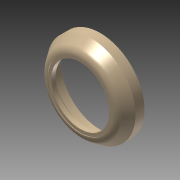
# Autodesk Inventor part: body
Saved by Autodesk Inventor 2015 SP1 (Build 190203100, 203)
## iProperties
Created: 2015-02-16
Part Number: body
Material: Polyethylene, Low Density
Document SubType Name: Modeling
Designer: Jostein
Density: 0.894 g/cm^3
Appearance: Smooth - Off-White
Author: Jostein
Autodesk Inventor part; units mm, degrees
ref_plane "YZ Plane" through (0, 0, 0) normal (1, 0, 0) x (0, 1, 0)
ref_plane "XZ Plane" through (0, 0, 0) normal (0, 1, 0) x (-1, 0, 0)
ref_plane "XY Plane" through (0, 0, 0) normal (0, 0, 1) x (1, 0, 0)
sketch "Sketch1" plane through (0, 0, 0) normal (0, 0, 1) x (1, 0, 0)
  line L0 (-179, 3) -> (-179, 30)
  line L1 (-179, 30) -> (-199, 30)
  line L2 (-274, 126) -> (-244, 126)
  line L3 (-274, 126) -> (-274, 70)
  arc A0 (-239.9746, 21.3454) -> (-199, 0) centre (-199, 50) ccw
  line L4 (-274, 70) -> (-239.9746, 21.3454)
  line L5 (0, 0) -> (-199, 0) construction
  line L6 (-244, 126) -> (-244, 79.4492)
  line L7 (-244, 79.4492) -> (-215.3898, 38.5382)
  arc A1 (-215.3898, 38.5382) -> (-199, 30) centre (-199, 50) ccw
  line L8 (-179, 3) -> (-199, 3)
  line L9 (-199, 3) -> (-199, 0)
  line L10 (0, -31.2197) -> (0, 152.2033) construction
  line L11 (-239.9746, 21.3454) -> (-215.3898, 38.5382) construction
  dimension "d3" = 50
  dimension "d4" = 123
  dimension "d5" = 65
  dimension "d6" = 30
  dimension "d11" = 30
  dimension "d22" = 199
  dimension "d23" = 20
  dimension "d32" = 3
  dimension "d42" = 27
  dimension "d44" = 70
  constraints: 23 end point, 4 point on circle, 4 tangent, 3 horizontal, 3 perpendicular, 3 vertical, 2 centre point, 1 horizontal alignment, 1 parallel, 1 vertical alignment
  measures "d3" radius of A0
  measures "d4" vertical distance of L2.end L0.start
  measures "d5" horizontal distance of L2.end L0.end
  measures "d6" distance of L2.start L2.end
  measures "d11" distance between parallel lines of L4 L7
  measures "d22" distance of L5.end L5.start
  measures "d23" distance of L0.start L8.end
  measures "d32" distance of L8.end L5.end
  measures "d42" distance of L0.start L0.end
  measures "d44" vertical distance of L3.end L5.end
revolve "Revolution1" add sketch "Sketch1" angle 360 about axis through (0, -10, 0) along (0, 1, 0)
chamfer "Chamfer1" distance 5 angle 45 1 edges at (179, 30, 0)
body "Solid1"
